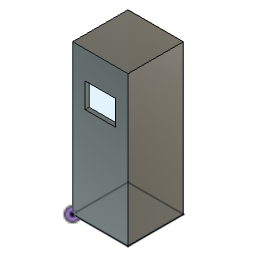
Waterproofing - soldered board case (Autodesk Fusion 360 design; units mm, degrees)
Autodesk Fusion 360 part; units mm, degrees
sketch "Sketch1" plane through (0, 0, 0) normal (0, 0, 1) x (1, 0, 0)
  line L0 (0, 0) -> (40, 0)
  line L1 (40, 0) -> (40, 40)
  line L2 (40, 40) -> (0, 40)
  line L3 (0, 40) -> (0, 0)
  dimension "d1" = 40
  dimension "d2" = 40
  constraint horizontal L0
  constraint vertical L1
  constraint horizontal L2
  constraint vertical L3
  constraint coincident L0.start L3.end
  measures "d1" distance of L0.start L2.end
  measures "d2" distance of L0.start L0.end
sketch "Sketch2" plane through (0, 0, 0) normal (0, 0, 1) x (1, 0, 0)
  circle A0 centre (10, 31) radius 3
  circle A1 centre (30, 31) radius 3
  circle A2 centre (10, 10) radius 3
  circle A3 centre (30, 11) radius 3
  line L0 (0, 40) -> (0, 0)
  line L1 (40, 0) -> (40, 40)
  line L2 (40, 40) -> (0, 40)
  line L3 (0, 0) -> (40, 0)
  dimension "d3" = 6
  dimension "d4" = 6
  dimension "d5" = 6
  dimension "d6" = 6
  dimension "d7" = 10
  dimension "d8" = 10
  dimension "d9" = 10
  dimension "d10" = 10
  dimension "d11" = 9
  dimension "d12" = 9
  dimension "d13" = 10
  dimension "d14" = 11
  measures "d3" diameter of A0
  measures "d4" diameter of A1
  measures "d5" diameter of A2
  measures "d6" diameter of A3
  measures "d7" distance of A0.centre L0
  measures "d8" distance of A1.centre L1
  measures "d9" distance of A3.centre L1
  measures "d10" distance of A2.centre L0
  measures "d11" distance of A0.centre L2
  measures "d12" distance of A1.centre L2
  measures "d13" distance of A2.centre L3
  measures "d14" distance of A3.centre L3
extrude "Extrude1" add sketch "Sketch2" along normal blind 3
sketch "Sketch3" plane through (0, 0, 3) normal (0, 0, 1) x (-1, 0, 0)
  circle A0 centre (-30, -31) radius 3
  circle A1 centre (-30, -11) radius 3
  circle A2 centre (-10, -31) radius 3
  circle A3 centre (-10, -10) radius 3
  line L0 (0, 0) -> (-40, 0)
  line L1 (-40, 0) -> (-40, -40)
  line L2 (-40, -40) -> (0, -40)
  line L3 (0, -40) -> (0, 0)
  circle A4 centre (-10, -31) radius 4.3
  circle A5 centre (-30, -31) radius 4.3
  circle A6 centre (-10, -10) radius 4.3
  circle A7 centre (-30, -11) radius 4.3
  line L4 (0, -40) -> (-40, -40)
  line L5 (-40, -40) -> (-40, 0)
  line L6 (-40, 0) -> (0, 0)
  line L7 (0, 0) -> (0, -40)
  dimension "d17" = 8.6
  dimension "d18" = 8.6
  dimension "d19" = 8.6
  dimension "d20" = 8.6
  constraint concentric A2 A4
  constraint concentric A0 A5
  constraint concentric A3 A6
  constraint concentric A1 A7
  constraint horizontal L4
  constraint vertical L5
  constraint horizontal L6
  constraint vertical L7
  constraint coincident L0.end L1.start
  constraint coincident L2.end L3.start
  measures "d17" diameter of A4
  measures "d18" diameter of A5
  measures "d19" diameter of A6
  measures "d20" diameter of A7
extrude "Extrude2" add sketch "Sketch3" along normal blind 5 contours L0 L1 L2 L3 L4 L5 L6 L7
sketch "Sketch4" plane through (0, 0, 8) normal (0, 0, 1) x (-1, 0, 0)
  circle A0 centre (-30, -11) radius 4.3
  circle A1 centre (-30, -31) radius 4.3
  circle A2 centre (-10, -31) radius 4.3
  circle A3 centre (-10, -10) radius 4.3
  line L0 (0, 0) -> (-40, 0)
  line L1 (-40, 0) -> (-40, -40)
  line L2 (-40, -40) -> (0, -40)
  line L3 (0, -40) -> (0, 0)
  line L4 (-40, -40) -> (-37, -40)
  line L5 (-37, -40) -> (-37, 0)
  line L6 (-37, 0) -> (-40, 0)
  line L7 (-40, 0) -> (-40, -40)
  line L8 (0, -40) -> (-3, -40)
  line L9 (-3, -40) -> (-3, 0)
  line L10 (-3, 0) -> (0, 0)
  line L11 (0, 0) -> (0, -40)
  line L12 (0, -40) -> (-40, -40)
  line L13 (-40, -40) -> (-40, -37)
  line L14 (-40, -37) -> (0, -37)
  line L15 (0, -37) -> (0, -40)
  line L16 (0, 0) -> (-40, 0)
  line L17 (-40, 0) -> (-40, -3)
  line L18 (-40, -3) -> (0, -3)
  line L19 (0, -3) -> (0, 0)
  dimension "d23" = 3
  dimension "d24" = 40
  dimension "d25" = 3
  dimension "d26" = 3
  dimension "d27" = 3
  constraint horizontal L4
  constraint vertical L5
  constraint horizontal L6
  constraint vertical L7
  constraint coincident L0 L5.end
  constraint coincident L1.end L2.start
  constraint horizontal L8
  constraint vertical L9
  constraint horizontal L10
  constraint vertical L11
  constraint coincident L2.end L3.start
  constraint horizontal L12
  constraint vertical L13
  constraint horizontal L14
  constraint vertical L15
  constraint horizontal L16
  constraint vertical L17
  constraint horizontal L18
  constraint vertical L19
  constraint coincident L0.start L3.end
  measures "d23" distance of L5.end L0.end
  measures "d24" distance of L2.end L0.start
  measures "d25" distance of L9.end L0.start
  measures "d26" distance of L2.end L14.end
  measures "d27" distance of L0.start L18.end
extrude "Extrude3" add sketch "Sketch4" along normal blind 100 contours L0 L3 L9 L10 L11 L16 L18 L19 | L0 L5 L9 L16 L18 | L3 L9 L11 L14 L18 | L0 L1 L5 L6 L7 L16 L17 L18 | L2 L3 L8 L9 L11 L12 L14 L15 | L1 L5 L7 L14 L18 | L2 L5 L9 L12 L14 | L1 L2 L4 L5 L7 L12 L13 L14
sketch "Sketch5" plane through (0, 0, 0) normal (0, -1, 0) x (1, 0, 0)
  line L0 (0, 0) -> (40, 0)
  line L1 (40, 0) -> (40, 108)
  line L2 (40, 108) -> (0, 108)
  line L3 (0, 108) -> (0, 0)
sketch "Sketch6" plane through (0, 0, 0) normal (-1, 0, 0) x (0, -1, 0)
  line L0 (-40, 0) -> (0, 0)
  line L1 (0, 0) -> (0, 108)
  line L2 (0, 108) -> (-40, 108)
  line L3 (-40, 108) -> (-40, 0)
  line L4 (-3, 8) -> (-37, 8)
  line L5 (-37, 8) -> (-37, 98)
  line L6 (-37, 98) -> (-3, 98)
  line L7 (-3, 98) -> (-3, 8)
  line L8 (-40, 0) -> (0, 0)
  dimension "d30" = 3
  dimension "d31" = 3
  dimension "d32" = 8
  dimension "d33" = 90
  constraint horizontal L4
  constraint vertical L5
  constraint horizontal L6
  constraint vertical L7
  measures "d30" distance of L3 L5
  measures "d31" distance of L1 L7
  measures "d32" distance of L4 L8
  measures "d33" distance of L4.start L6.end
extrude "Extrude4" cut sketch "Sketch6" against normal blind 10 contours L4 L5 L6 L7
sketch "Sketch7" plane through (0, 0, 108) normal (0, 0, 1) x (-1, 0, 0)
  line L0 (-3, -3) -> (-3, -37)
  line L1 (-3, -37) -> (-37, -37)
  line L2 (-37, -37) -> (-37, -3)
  line L3 (-37, -3) -> (-3, -3)
  line L4 (0, -40) -> (0, 0)
  line L5 (0, 0) -> (-40, 0)
  line L6 (-40, 0) -> (-40, -40)
  line L7 (-40, -40) -> (0, -40)
  line L8 (-3, -37) -> (-37, -37)
  line L9 (-37, -37) -> (-37, -3)
  line L10 (-37, -3) -> (-3, -3)
  line L11 (-3, -3) -> (-3, -37)
  constraint horizontal L8
  constraint vertical L9
  constraint horizontal L10
  constraint vertical L11
  constraint coincident L2.end L3.start
  constraint coincident L0.end L1.start
extrude "Extrude5" add sketch "Sketch7" against normal blind 3 contours L0 L1 L2 L3 L8 L9 L10 L11
sketch "Sketch8" plane through (0, 0, 0) normal (0, -1, 0) x (1, 0, 0)
  line L0 (9, 88) -> (31, 88)
  line L1 (31, 88) -> (31, 70)
  line L2 (31, 70) -> (9, 70)
  line L3 (9, 70) -> (9, 88)
  line L4 (0, 108) -> (0, 0)
  line L5 (40, 0) -> (40, 108)
  line L6 (40, 108) -> (0, 108)
  line L7 (0, 0) -> (40, 0)
  dimension "d38" = 9
  dimension "d39" = 9
  dimension "d40" = 20
  dimension "d41" = 70
  constraint horizontal L0
  constraint vertical L1
  constraint horizontal L2
  constraint vertical L3
  measures "d38" distance of L3 L4
  measures "d39" distance of L1 L5
  measures "d40" distance of L0 L6
  measures "d41" distance of L2 L7
extrude "Extrude6" cut sketch "Sketch8" against normal blind 15 contours L0 L1 L2 L3
sketch "Sketch9" plane through (0, 0, 0) normal (-1, 0, 0) x (0, -1, 0)
  line L0 (-37, 8) -> (-37, 98)
  line L1 (-37, 98) -> (-3, 98)
  line L2 (-3, 98) -> (-3, 8)
  line L3 (-3, 8) -> (-37, 8)
  line L4 (-40, 0) -> (0, 0)
  line L5 (0, 0) -> (0, 108)
  line L6 (0, 108) -> (-40, 108)
  line L7 (-40, 108) -> (-40, 0)
